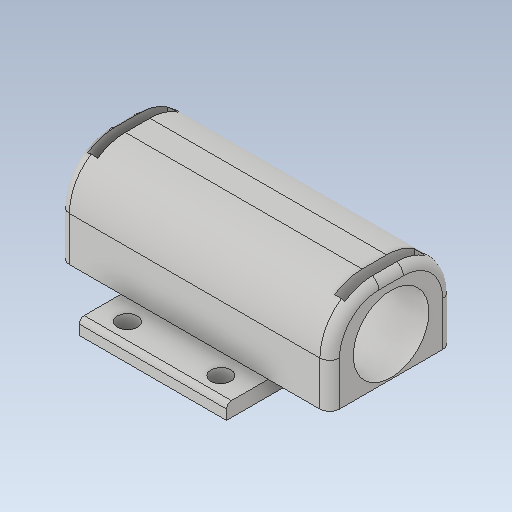
# Autodesk Inventor part: slave-slider-house
Saved by Autodesk Inventor 2020 (Build 240168000, 168)
## iProperties
Created: 2017-10-14
Part Number: slave-slider-house
Material: 一般
Document SubType Name: Modeling
Designer: wangh
Density: 1 g/cm^3
Appearance: 默认值
Mass: 16.7492 g
Surface Area: 90.9685 cm^2
Volume: 16.7492 cm^3
Author: wangh
Autodesk Inventor part; units mm, degrees
ref_plane "YZ Plane" through (0, 0, 0) normal (1, 0, 0) x (0, 1, 0)
ref_plane "XZ Plane" through (0, 0, 0) normal (0, 1, 0) x (-1, 0, 0)
sketch "Sketch1" plane through (0, 0, 0) normal (0, 1, 0) x (-1, 0, 0)
  line L0 (-15, 21) -> (15, 21)
  line L1 (15, 21) -> (15, -21)
  line L2 (15, -21) -> (-15, -21)
  line L3 (-15, -21) -> (-15, 21)
  line L4 (-15, 21) -> (15, -21) construction
  line L5 (15, 21) -> (-15, -21) construction
  line L6 (-9.525, 16.6751) -> (9.525, 16.6751) construction
  line L7 (9.525, 16.6751) -> (9.525, -16.6751) construction
  line L8 (9.525, -16.6751) -> (-9.525, -16.6751) construction
  line L9 (-9.525, -16.6751) -> (-9.525, 16.6751) construction
  line L10 (-9.525, 16.6751) -> (9.525, -16.6751) construction
  line L11 (9.525, 16.6751) -> (-9.525, -16.6751) construction
  circle A0 centre (9.525, 16.6751) radius 2.032
  circle A1 centre (-9.525, -16.6751) radius 2.032
  circle A2 centre (9.525, -16.6751) radius 2.032
  circle A3 centre (-9.525, 16.6751) radius 2.032
  point P0 (0, 0)
  dimension "d0" = 30
  dimension "d1" = 42
  dimension "d2" = 33.3502
  dimension "d3" = 19.05
  dimension "d6" = 4.064
  dimension "d7" = 4.064
  dimension "d36" = 4.064
  dimension "d37" = 4.064
  constraints: 24 end point, 4 centre point, 4 coincident, 4 midpoint, 4 parallel, 2 horizontal, 2 perpendicular
  measures "d0" distance of L1.end L2.end
  measures "d1" distance of L0.end L1.end
  measures "d2" distance of L6.end L7.end
  measures "d3" distance of L6.start L6.end
  measures "d6" diameter of A0
  measures "d7" diameter of A1
  measures "d36" diameter of A2
  measures "d37" diameter of A3
extrude "Extrusion1" add sketch "Sketch1" against normal blind 3
sketch "Sketch2" plane through (0, 0, 0) normal (0, 1, 0) x (1, 0, 0)
  line L0 (27.5, -12.5) -> (-27.5, -12.5)
  line L1 (-27.5, -12.5) -> (-27.5, 12.5)
  line L2 (-27.5, 12.5) -> (27.5, 12.5)
  line L3 (27.5, 12.5) -> (27.5, -12.5)
  line L4 (27.5, -12.5) -> (-27.5, 12.5) construction
  line L5 (-27.5, -12.5) -> (27.5, 12.5) construction
  point P0 (0, 0)
  point P1 (0, 0)
  point P2 (0, 0)
  dimension "d9" = 25
  dimension "d13" = 55
  constraints: 12 end point, 3 midpoint, 2 parallel, 1 coincident, 1 horizontal, 1 perpendicular
  measures "d9" distance of L0.end L1.end
  measures "d13" distance of L1.end L2.end
extrude "Extrusion2" add sketch "Sketch2" along normal blind 19
sketch "Sketch3" plane through (27.5, 0, 12.5) normal (1, 0, 0) x (0, 0, -1)
  line L0 (25, 0) -> (0, 0) projected
  line L1 (25, 0) -> (25, 19) projected
  line L2 (0, 19) -> (25, 19) projected
  line L3 (0, 0) -> (0, 19) projected
  line L4 (33.5, 0) -> (25, 0) projected
  line L5 (25, 0) -> (0, 0) projected
  line L6 (0, 0) -> (-8.5, 0) projected
  line L7 (-8.5, 0) -> (-8.5, -3) projected
  line L8 (33.5, -3) -> (-8.5, -3) projected
  line L9 (33.5, 0) -> (33.5, -3) projected
  circle A0 centre (12.5, 8) radius 7.7
  point P0 (12.5, 0)
  point P1 (12.5, 0)
  point P2 (12.5, 0)
  dimension "d12" = 15.4
  dimension "d28" = 11
  constraints: 2 midpoint, 1 centre point, 1 vertical alignment
  measures "d12" diameter of A0
  measures "d28" distance from line of A0.centre L8
extrude "Extrusion3" cut sketch "Sketch3" against normal through all contours A0
fillet "Fillet1" radius 10 2 edges at (0, 19, -12.5) (0, 19, 12.5)
fillet "Fillet2" radius 2 10 edges at (27.5, 19, 0) (27.5, 16.0711, -9.5711) (27.5, 4.5, -12.5) (27.5, 4.5, 12.5) (27.5, 16.0711, 9.5711) (-27.5, 19, 0) (-27.5, 16.0711, 9.5711) (-27.5, 4.5, 12.5) (-27.5, 4.5, -12.5) (-27.5, 16.0711, -9.5711)
fillet "Fillet3" radius 1 2 edges at (0, 0, 21) (0, 0, -21)
sketch "Sketch4" plane through (0, 19, 0) normal (0, 1, 0) x (1, 0, 0)
  line L0 (26.2, -8.1) -> (24.1, -8.1)
  line L1 (24.1, -8.1) -> (24.1, 8.1)
  line L2 (24.1, 8.1) -> (26.2, 8.1)
  line L3 (26.2, 8.1) -> (26.2, -8.1)
  line L4 (25.5, -2.5) -> (-25.5, -2.5) projected
  line L5 (-25.5, 2.5) -> (25.5, 2.5) projected
  line L6 (-25.5, -2.5) -> (-25.5, 2.5) projected
  line L7 (25.5, 2.5) -> (25.5, -2.5) projected
  point P0 (0, 0)
  dimension "d16" = 24.1
  dimension "d18" = 2.1
  dimension "d34" = 8.1
  dimension "d35" = 8.1
  constraints: 8 end point, 2 parallel, 1 horizontal, 1 perpendicular
  measures "d16" distance from line of point (0, 0) L1
  measures "d18" distance between parallel lines of L1 L3
  measures "d34" vertical distance of point (0, 0) L0.end
  measures "d35" distance from line of point (0, 0) L2
extrude "Extrusion4" cut sketch "Sketch4" against normal blind 6.1 contours L0 L1 L4 L7 L5 L2 L3 | L1 L5 L7 L4
ref_plane "Work Plane1" through (0, 0, 10.5) normal (1, 0, 0) x (0, 0, -1)
mirror "Mirror1" about plane through (0, 0, 10.5) normal (1, 0, 0) of "Extrusion4"
sketch "Sketch5" plane through (0, 12.9, 0) normal (0, 1, 0) x (1, 0, 0)
  line L0 (26.2, 9.4632) -> (26.2, -9.4632) projected
  line L1 (24.1, -9.6414) -> (24.1, 9.6414) projected
  line L2 (-24.1, 9.6414) -> (-24.1, -9.6414) projected
  line L3 (-26.2, -9.4632) -> (-26.2, 9.4632) projected
  line L4 (26.2, -9.5) -> (24.1, -9.5)
  line L5 (24.1, -9.5) -> (24.1, 9.5)
  line L6 (24.1, 9.5) -> (26.2, 9.5)
  line L7 (26.2, 9.5) -> (26.2, -9.5)
  line L8 (-24.1, -9.5) -> (-26.2, -9.5)
  line L9 (-26.2, -9.5) -> (-26.2, 9.5)
  line L10 (-26.2, 9.5) -> (-24.1, 9.5)
  line L11 (-24.1, 9.5) -> (-24.1, -9.5)
  line L12 (-25.5, 9.6414) -> (-24.1, 9.6414) projected
  line L13 (-24.1, -9.6414) -> (-25.5, -9.6414) projected
  line L14 (-25.5, 9.6414) -> (-24.1, 9.6414) projected
  line L15 (-24.1, -9.6414) -> (-25.5, -9.6414) projected
  line L16 (24.1, 9.6414) -> (25.5, 9.6414) projected
  line L17 (24.1, -9.6414) -> (24.1, 9.6414) projected
  line L18 (25.5, -9.6414) -> (24.1, -9.6414) projected
  line L19 (26.2, 9.4632) -> (26.2, -9.4632) projected
  line L20 (24.1, 9.6414) -> (25.5, 9.6414) projected
  line L21 (25.5, -9.6414) -> (24.1, -9.6414) projected
  line L22 (-24.1, 9.6414) -> (-24.1, -9.6414) projected
  line L23 (-26.2, -9.4632) -> (-26.2, 9.4632) projected
  point P0 (0, 0)
  constraints: 16 end point, 4 parallel, 4 point on line, 2 horizontal, 2 perpendicular, 8 other
body "Solid1"
